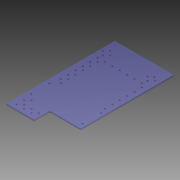
# Autodesk Inventor part: Electronics Board NXT
Saved by Autodesk Inventor 2014 SP2 (Build 180246200, 246)
## iProperties
Created: 2014-10-22
Part Number: Electronics Board NXT
Material: ABS Plastic
Document SubType Name: Modeling
Designer: Allison
Density: 1.06 g/cm^3
Appearance: Smooth - White
Author: Allison
Autodesk Inventor part; units mm, degrees
ref_plane "YZ Plane" through (0, 0, 0) normal (1, 0, 0) x (0, 1, 0)
ref_plane "XZ Plane" through (0, 0, 0) normal (0, 1, 0) x (-1, 0, 0)
ref_plane "XY Plane" through (0, 0, 0) normal (0, 0, 1) x (1, 0, 0)
sketch "Sketch1" plane through (0, 0, 0) normal (0, 1, 0) x (-1, 0, 0)
  arc A0 (334.15, 5.5) -> (337.85, 5.5) centre (336, 5.5) ccw
  arc A1 (345.85, 13.5) -> (342.15, 13.5) centre (344, 13.5) ccw
  arc A2 (329.85, 13.5) -> (326.15, 13.5) centre (328, 13.5) ccw
  arc A3 (328.4931, 19.1569) -> (332.1931, 19.1569) centre (330.3431, 19.1569) ccw
  arc A4 (334.15, 21.5) -> (337.85, 21.5) centre (336, 21.5) ccw
  arc A5 (332, 13.5) -> (340, 13.5) centre (336, 13.5) ccw
  arc A6 (337.85, 181.5) -> (334.15, 181.5) centre (336, 181.5) ccw
  arc A7 (334.15, 197.5) -> (337.85, 197.5) centre (336, 197.5) ccw
  arc A8 (340, 189.5) -> (332, 189.5) centre (336, 189.5) ccw
  arc A9 (329.85, 189.5) -> (326.15, 189.5) centre (328, 189.5) ccw
  arc A10 (345.85, 189.5) -> (342.15, 189.5) centre (344, 189.5) ccw
  line L0 (352, 176) -> (352, 203)
  arc A11 (244, 13.5) -> (236, 13.5) centre (240, 13.5) ccw
  arc A12 (241.85, 21.5) -> (238.15, 21.5) centre (240, 21.5) ccw
  arc A13 (244, 189.5) -> (236, 189.5) centre (240, 189.5) ccw
  arc A14 (233.85, 189.5) -> (230.15, 189.5) centre (232, 189.5) ccw
  line L1 (228.8458, 84.7173) -> (228.8458, 88.629)
  arc A15 (336, 137.5) -> (336, 145.5) centre (336, 141.5) ccw
  arc A16 (336, 121.5) -> (336, 129.5) centre (336, 125.5) ccw
  arc A17 (336, 105.5) -> (336, 113.5) centre (336, 109.5) ccw
  arc A18 (336, 89.5) -> (336, 97.5) centre (336, 93.5) ccw
  arc A19 (336, 73.5) -> (336, 81.5) centre (336, 77.5) ccw
  arc A20 (336, 57.5) -> (336, 65.5) centre (336, 61.5) ccw
  arc A21 (336, 41.5) -> (336, 49.5) centre (336, 45.5) ccw
  arc A22 (336, 25.5) -> (336, 33.5) centre (336, 29.5) ccw
  arc A23 (336, 153.5) -> (336, 161.5) centre (336, 157.5) ccw
  arc A24 (336, 169.5) -> (336, 177.5) centre (336, 173.5) ccw
  arc A25 (260, 189.5) -> (252, 189.5) centre (256, 189.5) ccw
  arc A26 (276, 189.5) -> (268, 189.5) centre (272, 189.5) ccw
  arc A27 (292, 189.5) -> (284, 189.5) centre (288, 189.5) ccw
  arc A28 (308, 189.5) -> (300, 189.5) centre (304, 189.5) ccw
  arc A29 (324, 189.5) -> (316, 189.5) centre (320, 189.5) ccw
  line L2 (352, 203) -> (228.8458, 203)
  line L3 (228.8458, 203) -> (228.8458, 0)
  line L4 (228.8458, 0) -> (352, 0)
  line L5 (352, 0) -> (352, 203)
  line L6 (-2.54, -2.54) -> (116.84, -2.54)
  line L7 (116.84, -2.54) -> (116.84, 193.04)
  line L8 (116.84, 193.04) -> (-2.54, 193.04)
  line L9 (-2.54, 193.04) -> (-2.54, -2.54)
  line L10 (-2.54, 95.25) -> (-2.54, 183.2483)
  line L11 (-2.54, 183.2483) -> (116.84, 183.2483)
  line L12 (-2.54, 183.2483) -> (-2.54, 7.2517)
  line L13 (-2.54, 7.2517) -> (116.84, 7.2517)
  line L14 (116.84, 183.2483) -> (100.838, 183.2483)
  line L15 (100.838, 183.2483) -> (100.838, 7.2517)
  circle A30 centre (100.838, 183.2483) radius 4.0005
  circle A31 centre (84.836, 183.2483) radius 4.0005
  circle A32 centre (68.834, 183.2483) radius 4.0005
  circle A33 centre (52.832, 183.2483) radius 4.0005
  circle A34 centre (36.83, 183.2483) radius 4.0005
  circle A35 centre (20.828, 183.2483) radius 4.0005
  circle A36 centre (4.826, 183.2483) radius 4.0005
  line L16 (100.838, 183.2483) -> (100.838, 175.2473)
  circle A37 centre (100.838, 175.2473) radius 1.8542
  line L17 (100.838, 183.2483) -> (104.5464, 183.2483)
  line L18 (100.838, 183.2483) -> (108.839, 183.2483)
  circle A38 centre (108.839, 183.2483) radius 1.8542
  point P0 (287.9997, 29.5)
  point P1 (228.8458, 85.5356)
  dimension "d0" = 203
  dimension "d1" = 123.1542
  dimension "d2" = 119.38
  dimension "d3" = 195.58
  dimension "d4" = 87.9983
  dimension "d5" = 175.9966
  dimension "d6" = 16.002
  dimension "d7" = 8.001
  dimension "d10" = 16.002
  dimension "d15" = 8.001
  dimension "d16" = 3.7084
  dimension "d17" = 3.7084
  dimension "d18" = 8.001
  dimension "d19" = 3.7084
  constraints: 60 point on circle, 39 centre point, 38 end point, 8 point on line, 5 perpendicular, 4 parallel, 3 coincident, 3 horizontal, 2 midpoint, 12 other
  measures "d0" distance of L2.end L3.end
  measures "d1" distance of L3.end L4.end
  measures "d2" distance of L8.end L7.end
  measures "d3" distance of L7.end L6.end
  measures "d4" distance of L10.start L10.end
  measures "d5" distance of L10.end L12.end
  measures "d6" distance of L11.end L14.end
  measures "d7" diameter of A30
  measures "d10" distance of L16.start A31.centre
  measures "d15" distance of L16.start L16.end
  measures "d16" diameter of A37
  measures "d17" distance of L16.start L17.end
  measures "d18" distance of L16.start L18.end
  measures "d19" diameter of A38
extrude "Extrusion1" add sketch "Sketch1" along normal blind 3.175 contours L9 L13 L7 L6 | L9 L11 A36 A35 A34 A33 A32 A31 A30 L15 A37 L13 | L13 L15 A37 A30 L11 A38 L7 | L11 A38 A30 A31 A32 A33 A34 A35 A36 L9 L8 L7 | A37 L15 | L15 A37 | A38 L11 | L11 A38 | A36 L11 | L11 A36 | A30 L11 L15 | L15 L11 A30 | L11 A30 | A35 L11 | L11 A35 | A31 L11 | L11 A31 | A34 L11 | L11 A34 | A32 L11 | L11 A32 | A33 L11 | L11 A33
extrude "Extrusion2" cut sketch "Sketch1" along normal blind 3.175 contours A37 L15 | L15 A37 | A38 L11 | L11 A38
pattern_linear "Rectangular Pattern1" count 7 spacing 16.002 along (1, 0, 0) of "Extrusion2"
pattern_linear "Rectangular Pattern2" count 12 spacing 16.002 along (0, 0, -1) of "Extrusion2"
sketch "Sketch2" plane through (0, 3.175, 0) normal (0, 1, 0) x (1, 0, 0)
  arc A0 (-101.4053, 2.54) -> (-100.2707, 2.54) centre (-100.838, 0.7747) ccw projected
  line L0 (2.54, 2.54) -> (-100.2707, 2.54) projected
  line L1 (-101.4053, 2.54) -> (-100.2707, 2.54)
  point P0 (0, 0)
  constraints: 2 end point, 1 collinear
extrude "Extrusion3" add sketch "Sketch2" against normal up to surface (3.175 mm away)
sketch "Sketch3" plane through (0, 3.175, 0) normal (0, 1, 0) x (1, 0, 0)
  line L0 (2.54, 2.54) -> (-116.84, 2.54) projected
  circle A0 centre (-108.839, -7.2263) radius 1.8542 projected
  circle A1 centre (-100.838, -15.2273) radius 1.8542 projected
  circle A2 centre (-108.839, -7.2263) radius 1.8542
  circle A3 centre (-100.838, -15.2273) radius 1.8542
  circle A4 centre (-92.837, -7.2263) radius 1.8542
  circle A5 centre (-84.836, -15.2273) radius 1.8542
  circle A6 centre (-76.835, -7.2263) radius 1.8542
  circle A7 centre (-68.834, -15.2273) radius 1.8542
  circle A8 centre (-60.833, -7.2263) radius 1.8542
  circle A9 centre (-52.832, -15.2273) radius 1.8542
  circle A10 centre (-44.831, -7.2263) radius 1.8542
  circle A11 centre (-36.83, -15.2273) radius 1.8542
  circle A12 centre (-28.829, -7.2263) radius 1.8542
  circle A13 centre (-20.828, -15.2273) radius 1.8542
  circle A14 centre (-12.827, -7.2263) radius 1.8542
  circle A15 centre (-4.826, -15.2273) radius 1.8542
  point P0 (0, 0)
  dimension "d34" = 16.002
  constraints: 14 centre point, 14 coincident, 2 concentric, 1 horizontal, 36 other
  measures "d34" distance of A3.centre A5.centre
extrude "Extrusion4" cut sketch "Sketch3" against normal blind 3.175 contours A4 | A5 | A6 | A7 | A8 | A9 | A10 | A11 | A12 | A13 | A14 | A15
sketch "Sketch4" plane through (0, 3.175, 0) normal (0, 1, 0) x (1, 0, 0)
  circle A0 centre (-36.83, -15.2273) radius 1.8542 projected
  circle A1 centre (-52.832, -15.2273) radius 1.8542 projected
  circle A2 centre (-68.834, -15.2273) radius 1.8542 projected
  line L0 (2.54, -193.04) -> (2.54, 2.54) projected
  circle A3 centre (-36.83, -175.2473) radius 1.8542 projected
  circle A4 centre (-52.832, -175.2473) radius 1.8542 projected
  circle A5 centre (-68.834, -175.2473) radius 1.8542 projected
  line L1 (-68.834, -175.2473) -> (-68.834, -15.2273)
  line L2 (-68.834, -15.2273) -> (-52.832, -15.2273)
  line L3 (-52.832, -15.2273) -> (-52.832, -175.2473)
  line L4 (-52.832, -175.2473) -> (-36.83, -175.2473)
  line L5 (-36.83, -175.2473) -> (-36.83, -15.2273)
  circle A6 centre (-68.834, -95.2373) radius 1.8542
  circle A7 centre (-52.832, -95.2373) radius 1.8542
  circle A8 centre (-36.83, -95.2373) radius 1.8542
  point P0 (0, 0)
  dimension "d41" = 3.7084
  dimension "d42" = 3.7084
  dimension "d43" = 3.7084
  constraints: 10 end point, 4 parallel, 3 centre point, 3 midpoint, 1 perpendicular
  measures "d41" diameter of A6
  measures "d42" diameter of A7
  measures "d43" diameter of A8
extrude "Extrusion5" cut sketch "Sketch4" against normal blind 25.4 contours A6 L1 | L1 A6 | A7 L3 | L3 A7 | A8 L5 | L5 A8
sketch "Sketch5" plane through (0, 3.175, 0) normal (0, 1, 0) x (1, 0, 0)
  circle A0 centre (-4.826, -159.2453) radius 1.8542
  point P0 (0, 0)
  dimension "d46" = 3.7084
  constraints: 1 centre point
  measures "d46" diameter of A0
extrude "Extrusion6" cut sketch "Sketch5" against normal blind 25.4
pattern_linear "Rectangular Pattern3" count 9 spacing 16.002 along (0, 0, -1) of "Extrusion6"
sketch "Sketch6" plane through (0, 3.175, 0) normal (0, 1, 0) x (1, 0, 0)
  circle A0 centre (-4.826, -175.2473) radius 1.8542 projected
  circle A1 centre (-12.827, -183.2483) radius 1.8542 projected
  circle A2 centre (-20.828, -175.2473) radius 1.8542 projected
  line L0 (2.54, -193.04) -> (-28.829, -193.04)
  line L1 (-28.829, -193.04) -> (-28.829, -159.2453)
  line L2 (-28.829, -159.2453) -> (2.54, -159.2453)
  line L3 (2.54, -159.2453) -> (2.54, -193.04)
  point P0 (0, 0)
  constraints: 8 end point, 2 parallel, 1 horizontal, 1 perpendicular
extrude "Extrusion7" cut sketch "Sketch6" against normal blind 25.4
sketch "Sketch7" plane through (0, 3.175, 0) normal (0, 1, 0) x (1, 0, 0)
  circle A0 centre (-36.83, -95.2373) radius 1.8542 projected
  circle A1 centre (-68.834, -95.2373) radius 1.8542 projected
  circle A2 centre (-52.832, -95.2373) radius 1.8542 projected
  point P0 (0, 0)
extrude "Extrusion8" add sketch "Sketch7" against normal up to surface (3.175 mm away)
sketch "Sketch8" plane through (0, 0, 0) normal (0, -1, 0) x (1, 0, 0)
  arc A0 (-28.829, 185.1025) -> (-28.829, 181.3941) centre (-28.829, 183.2483) ccw projected
  arc A1 (-6.6802, 159.2453) -> (-2.9718, 159.2453) centre (-4.826, 159.2453) ccw projected
  line L0 (-28.829, 193.04) -> (-28.829, 159.2453)
  line L1 (-28.829, 159.2453) -> (2.54, 159.2453)
  arc A2 (-6.6802, 159.2453) -> (-2.9718, 159.2453) centre (-4.826, 159.2453) ccw
  arc A3 (-28.829, 185.1025) -> (-28.829, 181.3941) centre (-28.829, 183.2483) ccw
  point P0 (0, 0)
  constraints: 4 end point, 4 point on circle, 4 point on line, 2 centre point, 2 coincident, 1 perpendicular
extrude "Extrusion9" add sketch "Sketch8" against normal up to surface (3.175 mm away)
sketch "Sketch9" plane through (0, 3.175, 0) normal (0, 1, 0) x (1, 0, 0)
  circle A0 centre (-52.832, -175.2473) radius 1.8542 projected
  circle A1 centre (-44.831, -183.2483) radius 1.8542 projected
  circle A2 centre (-36.83, -175.2473) radius 1.8542 projected
  line L0 (-116.84, -193.04) -> (-28.829, -193.04) projected
  line L1 (-60.833, -193.04) -> (-28.829, -193.04)
  line L2 (-28.829, -193.04) -> (-28.829, -159.2453)
  line L3 (-28.829, -159.2453) -> (-60.833, -159.2453)
  line L4 (-60.833, -159.2453) -> (-60.833, -193.04)
  point P0 (0, 0)
  constraints: 8 end point, 2 parallel, 1 horizontal, 1 perpendicular, 1 point on line
extrude "Extrusion10" cut sketch "Sketch9" against normal blind 25.4
sketch "Sketch10" plane through (0, 3.175, 0) normal (0, 1, 0) x (1, 0, 0)
  arc A0 (-60.833, -181.3941) -> (-60.833, -185.1025) centre (-60.833, -183.2483) ccw projected
  line L0 (-116.84, -193.04) -> (-60.833, -193.04) projected
  line L1 (-60.833, -181.3941) -> (-60.833, -185.1025)
  point P0 (0, 0)
  constraints: 2 end point, 1 perpendicular
extrude "Extrusion11" add sketch "Sketch10" against normal up to surface (3.175 mm away)
fillet "Fillet1" radius 3.175 1 edges at (-60.833, 1.5875, 159.2453)
sketch "Sketch11" plane through (0, 3.175, 0) normal (0, 1, 0) x (1, 0, 0)
  circle A0 centre (-112.8662, -107.914) radius 1.8542
  circle A1 centre (-1.1898, -107.914) radius 1.8542
  circle A2 centre (-1.1898, -147.7728) radius 1.8542
  circle A3 centre (-112.8662, -147.7728) radius 1.8542
  point P0 (0, 0)
  dimension "d63" = 3.7084
  dimension "d64" = 3.7084
  dimension "d65" = 3.7084
  dimension "d66" = 3.7084
  constraints: 4 centre point
  measures "d63" diameter of A0
  measures "d64" diameter of A1
  measures "d65" diameter of A2
  measures "d66" diameter of A3
extrude "Extrusion12" cut sketch "Sketch11" against normal blind 25.4
sketch "Sketch12" plane through (0, 3.175, 0) normal (0, 1, 0) x (1, 0, 0)
  circle A0 centre (-108.839, -151.2443) radius 1.8542 projected
  circle A1 centre (-100.838, -143.2433) radius 1.8542 projected
  circle A2 centre (-108.839, -135.2423) radius 1.8542 projected
  circle A3 centre (-100.838, -127.2413) radius 1.8542 projected
  circle A4 centre (-108.839, -119.2403) radius 1.8542 projected
  circle A5 centre (-100.838, -111.2393) radius 1.8542 projected
  circle A6 centre (-108.839, -103.2383) radius 1.8542 projected
  circle A7 centre (-4.826, -143.2433) radius 1.8542 projected
  circle A8 centre (-4.826, -127.2413) radius 1.8542 projected
  circle A9 centre (-4.826, -111.2393) radius 1.8542 projected
  point P0 (0, 0)
extrude "Extrusion13" add sketch "Sketch12" against normal up to surface (3.175 mm away)
sketch "Sketch13" plane through (0, 3.175, 0) normal (0, 1, 0) x (1, 0, 0)
  line L0 (-116.84, 2.54) -> (2.54, 2.54)
  line L1 (2.54, 2.54) -> (2.54, 43.2395)
  line L2 (2.54, 43.2395) -> (-116.84, 43.2395)
  line L3 (-116.84, 43.2395) -> (-116.84, 2.54)
  point P0 (0, 0)
  constraints: 8 end point, 2 parallel, 1 horizontal, 1 perpendicular
extrude "Extrusion14" add sketch "Sketch13" against normal up to surface (3.175 mm away)
sketch "Sketch14" plane through (0, 3.175, 0) normal (0, 1, 0) x (1, 0, 0)
  circle A0 centre (-12.827, -7.2263) radius 1.8542 projected
  circle A1 centre (-28.829, -7.2263) radius 1.8542 projected
  circle A2 centre (-44.831, -7.2263) radius 1.8542 projected
  circle A3 centre (-60.833, -7.2263) radius 1.8542 projected
  circle A4 centre (-76.835, -7.2263) radius 1.8542 projected
  circle A5 centre (-92.837, -7.2263) radius 1.8542 projected
  circle A6 centre (-84.836, -15.2273) radius 1.8542 projected
  circle A7 centre (-68.834, -15.2273) radius 1.8542 projected
  circle A8 centre (-52.832, -15.2273) radius 1.8542 projected
  circle A9 centre (-36.83, -15.2273) radius 1.8542 projected
  circle A10 centre (-20.828, -15.2273) radius 1.8542 projected
  point P0 (0, 0)
extrude "Extrusion15" add sketch "Sketch14" against normal up to surface (3.175 mm away)
sketch "Sketch15" plane through (0, 0, 0) normal (0, -1, 0) x (1, 0, 0)
  arc A0 (-115.8166, -12.8) -> (-115.7922, -9.3001) centre (-115.8044, -11.0501) ccw
  arc A1 (-115.7922, -9.3001) -> (-115.8166, -12.8) centre (-115.8044, -11.0501) ccw
  arc A2 (-99.7922, -9.3001) -> (-99.8166, -12.8) centre (-99.8044, -11.0501) ccw
  arc A3 (-99.8166, -12.8) -> (-99.7922, -9.3001) centre (-99.8044, -11.0501) ccw
  arc A4 (-19.0796, -9.9743) -> (-19.104, -13.4742) centre (-19.0918, -11.7242) ccw
  arc A5 (-19.104, -13.4742) -> (-19.0796, -9.9743) centre (-19.0918, -11.7242) ccw
  arc A6 (-3.0796, -9.9743) -> (-3.104, -13.4742) centre (-3.0918, -11.7242) ccw
  arc A7 (-3.104, -13.4742) -> (-3.0796, -9.9743) centre (-3.0918, -11.7242) ccw
  line L0 (2.54, 159.2453) -> (2.54, -43.2395) projected
  line L1 (-115.8044, -11.0501) -> (-99.8044, -11.0501)
  line L2 (-99.8044, -11.0501) -> (-107.8044, -11.0501)
  line L3 (-107.8044, -11.0501) -> (-107.8044, -3.0491)
  line L4 (-19.0918, -11.7242) -> (-3.0918, -11.7242)
  line L5 (-3.0918, -11.7242) -> (-11.0918, -11.7242)
  line L6 (-11.0918, -11.7242) -> (-11.0918, -3.7232)
  circle A8 centre (-107.8044, -3.0491) radius 1.8542
  circle A9 centre (-11.0918, -3.7232) radius 1.8542
  circle A10 centre (-107.8044, -19.0511) radius 1.8542
  circle A11 centre (-11.0918, -18.3769) radius 1.8542
  dimension "d86" = 8.001
  dimension "d87" = 8.001
  dimension "d88" = 3.7084
  dimension "d89" = 3.7084
  constraints: 16 point on circle, 12 centre point, 12 end point, 4 perpendicular, 2 coincident, 2 midpoint, 2 symmetric about line, 2 other
  measures "d86" distance of L2.end L3.end
  measures "d87" distance of L5.end L6.end
  measures "d88" diameter of A8
  measures "d89" diameter of A9
sketch "Sketch17" plane through (-116.84, 0, -43.2395) normal (-1, 0, 0) x (0, 0, 1)
  line L0 (236.2795, 0) -> (0, 0) projected
  line L1 (236.2795, 0) -> (236.2795, 3.175) projected
  line L2 (0, 3.175) -> (236.2795, 3.175) projected
  line L3 (0, 3.175) -> (0, 0) projected
  point P0 (43.2395, 0)
extrude "Extrusion18" add sketch "Sketch17" along normal blind 5.08
extrude "Extrusion19" cut sketch "Sketch15" against normal blind 127
sketch "Sketch18" plane through (0, 0, 0) normal (0, -1, 0) x (1, 0, 0)
  line L0 (2.54, 159.2453) -> (-57.658, 159.2453) projected
  circle A0 centre (-108.839, 7.2263) radius 1.8542 projected
  line L1 (-108.839, 7.2263) -> (-92.837, 7.2263)
  circle A1 centre (-92.837, 7.2263) radius 1.8542
  point P0 (0, 0)
  dimension "d92" = 16.002
  dimension "d93" = 3.7084
  constraints: 2 end point, 1 centre point, 1 coincident, 1 parallel
  measures "d92" distance of L1.start L1.end
  measures "d93" diameter of A1
extrude "Extrusion20" cut sketch "Sketch18" against normal blind 127 contours A1
pattern_linear "Rectangular Pattern4" count 6 spacing 16.002 along (1, 0, 0) of "Extrusion20"
sketch "Sketch19" plane through (2.54, 0, 159.2453) normal (1, 0, 0) x (0, 0, -1)
  line L0 (0, 3.175) -> (0, 0) projected
  line L1 (0, 0) -> (202.4848, 0) projected
  line L2 (202.4848, 3.175) -> (202.4848, 0) projected
  line L3 (0, 3.175) -> (202.4848, 3.175) projected
  point P0 (159.2453, 0)
extrude "Extrusion21" add sketch "Sketch19" along normal blind 3.81
body "Solid1"
